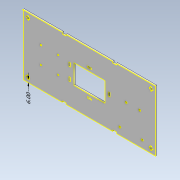
# Autodesk Inventor part: plate_2
Saved by Autodesk Inventor 2022 (Build 260153000, 153)
## iProperties
Created: 2023-04-28
Part Number: plate_2
Material: 一般
Document SubType Name: Modeling
Designer: Johnny Jou
Density: 1 g/cm^3
Appearance: 預設
Author: Johnny Jou
Autodesk Inventor part; units mm, degrees
ref_plane "YZ Plane" through (0, 0, 0) normal (1, 0, 0) x (0, 1, 0)
ref_plane "XZ Plane" through (0, 0, 0) normal (0, 1, 0) x (-1, 0, 0)
ref_plane "XY Plane" through (0, 0, 0) normal (0, 0, 1) x (1, 0, 0)
sketch "草圖1" plane through (0, 0, 0) normal (0, 0, 1) x (1, 0, 0)
  line L0 (0, 0) -> (284, 0)
  line L1 (284, 0) -> (284, -130)
  line L2 (284, -130) -> (0, -130)
  line L3 (0, -130) -> (0, 0)
  dimension "d0" = 284
  dimension "d1" = 130
  constraints: 8 end point, 2 parallel, 1 coincident, 1 horizontal, 1 perpendicular
  measures "d0" distance of L1.end L2.end
  measures "d1" distance of L0.end L1.end
extrude "擠出1" add sketch "草圖1" along normal blind 3
sketch "草圖2" plane through (0, 0, 3) normal (0, 0, 1) x (1, 0, 0)
  line L0 (35, -86.5) -> (78, -86.5)
  line L1 (78, -86.5) -> (78, -43.5)
  line L2 (78, -43.5) -> (35, -43.5)
  line L3 (35, -43.5) -> (35, -86.5)
  circle A0 centre (75, -46.5) radius 1.5
  circle A1 centre (38, -46.5) radius 1.5
  circle A2 centre (75, -83.5) radius 1.5
  circle A3 centre (38, -83.5) radius 1.5
  line L4 (0, 0) -> (0, -130) projected
  line L5 (284, 0) -> (0, 0) projected
  point P0 (74.3802, -81.4068)
  dimension "d44" = 35
  dimension "d45" = 43
  dimension "d46" = 43
  dimension "d47" = 3
  dimension "d48" = 3
  dimension "d49" = 3
  dimension "d50" = 3
  dimension "d51" = 3
  dimension "d52" = 3
  dimension "d53" = 3
  dimension "d54" = 3
  dimension "d55" = 3
  dimension "d56" = 43.5
  constraints: 8 end point, 4 centre point, 3 equal radius, 3 perpendicular
  measures "d44" distance between parallel lines of L4 L3
  measures "d45" distance of L1.end L2.end
  measures "d46" distance of L2.end L0.start
  measures "d47" distance from line of L2 A1.centre
  measures "d48" distance from line of L3 A1.centre
  measures "d49" distance from line of L2 A0.centre
  measures "d50" distance from line of L1 A0.centre
  measures "d51" distance from line of L1 A2.centre
  measures "d52" distance from line of L0 A2.centre
  measures "d53" distance from line of L3 A3.centre
  measures "d54" distance from line of L0 A3.centre
  measures "d55" diameter of A1
  measures "d56" distance between parallel lines of L5 L2
extrude "擠出2" cut sketch "草圖2" against normal up to surface (3 mm away) contours A0 | A1 | A2 | A3
sketch "草圖3" plane through (0, 0, 3) normal (0, 0, 1) x (1, 0, 0)
  line L0 (100.85, -42.4246) -> (100.85, -38)
  line L1 (183.15, -84.8295) -> (183.15, -92)
  line L2 (100.85, -38) -> (183.15, -38)
  line L3 (183.15, -38) -> (183.15, -92)
  line L4 (183.15, -92) -> (100.85, -92)
  line L5 (100.85, -92) -> (100.85, -38)
  line L6 (284, 0) -> (0, 0) projected
  line L7 (284, -130) -> (284, 0) projected
  line L8 (0, 0) -> (284, -130) construction
  line L9 (0, 0) -> (0, -130) projected
  line L10 (0, -130) -> (284, 0) construction
  line L11 (100.85, -38) -> (183.15, -92) construction
  line L12 (183.15, -38) -> (100.85, -92) construction
  line L13 (138, -35.05) -> (146, -35.05)
  line L14 (146, -35.05) -> (146, -38)
  line L15 (146, -38) -> (138, -38)
  line L16 (138, -38) -> (138, -35.05)
  line L17 (138, -92) -> (146, -92)
  line L18 (146, -92) -> (146, -94.95)
  line L19 (146, -94.95) -> (138, -94.95)
  line L20 (138, -94.95) -> (138, -92)
  line L21 (183.15, -61) -> (186.1, -61)
  line L22 (186.1, -61) -> (186.1, -69)
  line L23 (186.1, -69) -> (183.15, -69)
  line L24 (183.15, -69) -> (183.15, -61)
  line L25 (97.9, -48) -> (100.85, -48)
  line L26 (100.85, -48) -> (100.85, -56)
  line L27 (100.85, -56) -> (97.9, -56)
  line L28 (97.9, -56) -> (97.9, -48)
  line L29 (97.9, -75.1961) -> (100.85, -75.1961)
  line L30 (100.85, -75.1961) -> (100.85, -83.1961)
  line L31 (100.85, -83.1961) -> (97.9, -83.1961)
  line L32 (97.9, -83.1961) -> (97.9, -75.1961)
  point P0 (142, -65)
  point P1 (142, -35.05)
  point P2 (142, -65)
  point P3 (186.1, -65)
  point P4 (142, -65)
  dimension "d6" = 54
  dimension "d7" = 82.3
  dimension "d8" = 8
  dimension "d9" = 2.95
  dimension "d10" = 8
  dimension "d11" = 2.95
  dimension "d12" = 8
  dimension "d13" = 2.95
  dimension "d14" = 2.95
  dimension "d15" = 8
  dimension "d16" = 8
  dimension "d17" = 10
  constraints: 60 end point, 12 parallel, 6 horizontal, 6 midpoint, 6 perpendicular, 5 collinear, 2 point on line, 1 horizontal alignment, 1 vertical alignment
  measures "d6" distance between parallel lines of L4 L2
  measures "d7" distance between parallel lines of L5 L3
  measures "d8" distance of L18.end L19.end
  measures "d9" distance of L17.end L18.end
  measures "d10" distance of L13.start L13.end
  measures "d11" distance of L13.end L14.end
  measures "d12" distance of L21.end L22.end
  measures "d13" distance of L21.start L21.end
  measures "d14" distance of L25.start L25.end
  measures "d15" distance of L27.end L25.start
  measures "d16" distance of L31.end L29.start
  measures "d17" distance between parallel lines of L2 L25
extrude "擠出3" cut sketch "草圖3" against normal up to surface (3 mm away) contours L5 L27 L28 L25 | L16 L13 L14 L2 | L5 L31 L32 L29 | L21 L22 L23 L3 | L4 L18 L19 L20
sketch "草圖4" plane through (0, 0, 3) normal (0, 0, 1) x (1, 0, 0)
  line L0 (284, -130) -> (284, 0) projected
  circle A0 centre (249.8545, -61.6059) radius 2
  circle A1 centre (220.8545, -61.6059) radius 2
  circle A2 centre (207.3545, -114.1059) radius 2
  circle A3 centre (255.3545, -114.1059) radius 2
  point P0 (0, 0)
  point P1 (32.4, -26.5)
  dimension "d25" = 48
  dimension "d26" = 5.5
  dimension "d27" = 52.5
  dimension "d28" = 29
  dimension "d29" = 13.5
  dimension "d30" = 52.5
  constraints: 4 centre point
  measures "d25" distance of A3.centre A2.centre
  measures "d26" horizontal distance of A0.centre A3.centre
  measures "d27" vertical distance of A3.centre A0.centre
  measures "d28" distance of A0.centre A1.centre
  measures "d29" horizontal distance of A2.centre A1.centre
  measures "d30" vertical distance of A2.centre A1.centre
extrude "擠出4" cut sketch "草圖4" against normal blind 10
sketch "草圖5" plane through (0, 0, 3) normal (0, 0, 1) x (1, 0, 0)
  line L0 (84, 0) -> (92, 0)
  line L1 (92, 0) -> (92, -2.95)
  line L2 (92, -2.95) -> (84, -2.95)
  line L3 (84, -2.95) -> (84, 0)
  line L4 (192, 0) -> (200, 0)
  line L5 (200, 0) -> (200, -2.95)
  line L6 (200, -2.95) -> (192, -2.95)
  line L7 (192, -2.95) -> (192, 0)
  line L8 (192, -127.05) -> (200, -127.05)
  line L9 (200, -127.05) -> (200, -130)
  line L10 (200, -130) -> (192, -130)
  line L11 (192, -130) -> (192, -127.05)
  line L12 (84, -127.05) -> (92, -127.05)
  line L13 (92, -127.05) -> (92, -130)
  line L14 (92, -130) -> (84, -130)
  line L15 (84, -130) -> (84, -127.05)
  line L16 (284, 0) -> (0, 0) projected
  line L17 (0, -130) -> (284, -130) projected
  line L18 (0, 0) -> (0, -130) projected
  dimension "d33" = 2.95
  dimension "d34" = 8
  dimension "d36" = 2.95
  dimension "d37" = 8
  dimension "d38" = 100
  dimension "d39" = 8
  dimension "d43" = 84
  constraints: 32 end point, 9 collinear, 8 parallel, 4 horizontal, 4 perpendicular
  measures "d33" distance between parallel lines of L2 L0
  measures "d34" distance of L0.start L0.end
  measures "d36" distance between parallel lines of L14 L12
  measures "d37" distance of L13.end L14.end
  measures "d38" distance between parallel lines of L11 L13
  measures "d39" distance of L8.start L8.end
  measures "d43" distance between parallel lines of L18 L3
extrude "擠出5" cut sketch "草圖5" against normal up to surface (3 mm away)
sketch "草圖6" plane through (0, 0, 3) normal (0, 0, 1) x (1, 0, 0)
  line L0 (8.525, -6) -> (11.475, -6)
  line L1 (11.475, -6) -> (11.475, -14)
  line L2 (11.475, -14) -> (8.525, -14)
  line L3 (8.525, -14) -> (8.525, -6)
  line L4 (6, -8.525) -> (14, -8.525)
  line L5 (14, -8.525) -> (14, -11.475)
  line L6 (14, -11.475) -> (6, -11.475)
  line L7 (6, -11.475) -> (6, -8.525)
  line L8 (6, -8.525) -> (14, -11.475) construction
  line L9 (14, -8.525) -> (6, -11.475) construction
  line L10 (8.525, -14) -> (11.475, -6) construction
  line L11 (11.475, -14) -> (8.525, -6) construction
  line L12 (84, 0) -> (0, 0) construction
  line L13 (0, 0) -> (0, -130) construction
  point P0 (10, -10)
  point P1 (8.525, -11.475)
  point P2 (11.475, -11.475)
  point P3 (11.475, -8.525)
  point P4 (8.525, -8.525)
  dimension "d57" = 8
  dimension "d58" = 8
  dimension "d59" = 2.95
  dimension "d60" = 2.95
  dimension "d61" = 6
  dimension "d62" = 6
  constraints: 24 end point, 4 parallel, 2 horizontal, 2 midpoint, 2 perpendicular
  measures "d57" distance of L4.start L4.end
  measures "d58" distance of L0.end L1.end
  measures "d59" distance of L0.start L0.end
  measures "d60" distance of L4.end L5.end
  measures "d61" distance between parallel lines of L12 L0
  measures "d62" distance between parallel lines of L13 L7
extrude "擠出6" cut sketch "草圖6" against normal up to surface (3 mm away)
pattern_linear "矩形陣列1" count 2 spacing 110 along (0, -1, 0) count 2 spacing 264 along (1, 0, 0) of "擠出6"
sketch "草圖7" plane through (0, 0, 3) normal (0, 0, 1) x (1, 0, 0)
  line L0 (108.85, -44) -> (175.15, -44)
  line L1 (175.15, -44) -> (175.15, -86)
  line L2 (175.15, -86) -> (108.85, -86)
  line L3 (108.85, -86) -> (108.85, -44)
  line L4 (146, -38) -> (138, -38) projected
  line L5 (138, -92) -> (146, -92) projected
  line L6 (183.15, -69) -> (183.15, -61) projected
  line L7 (100.85, -48) -> (100.85, -56) projected
  point P0 (0, 0)
  dimension "d74" = 6
  dimension "d75" = 6
  dimension "d76" = 8
  dimension "d77" = 8
  constraints: 8 end point, 2 parallel, 1 horizontal, 1 perpendicular
  measures "d74" distance between parallel lines of L0 L4
  measures "d75" distance between parallel lines of L5 L2
  measures "d76" distance between parallel lines of L6 L1
  measures "d77" distance between parallel lines of L7 L3
extrude "擠出7" cut sketch "草圖7" against normal blind 10
sketch "草圖8" plane through (0, 0, 3) normal (0, 0, 1) x (1, 0, 0)
  line L0 (175.15, -44) -> (175.15, -86) projected
  line L1 (175.15, -86) -> (108.85, -86) projected
  line L2 (108.85, -86) -> (108.85, -44) projected
  line L3 (108.85, -44) -> (175.15, -44) projected
  line L4 (272.525, -116) -> (275.475, -116) projected
  line L5 (275.475, -116) -> (275.475, -118.525) projected
  line L6 (275.475, -118.525) -> (278, -118.525) projected
  line L7 (278, -118.525) -> (278, -121.475) projected
  line L8 (278, -121.475) -> (275.475, -121.475) projected
  line L9 (275.475, -121.475) -> (275.475, -124) projected
  line L10 (275.475, -124) -> (272.525, -124) projected
  line L11 (272.525, -124) -> (272.525, -121.475) projected
  line L12 (272.525, -121.475) -> (270, -121.475) projected
  line L13 (270, -121.475) -> (270, -118.525) projected
  line L14 (270, -118.525) -> (272.525, -118.525) projected
  line L15 (272.525, -118.525) -> (272.525, -116) projected
  line L16 (272.525, -6) -> (275.475, -6) projected
  line L17 (275.475, -6) -> (275.475, -8.525) projected
  line L18 (275.475, -8.525) -> (278, -8.525) projected
  line L19 (278, -8.525) -> (278, -11.475) projected
  line L20 (278, -11.475) -> (275.475, -11.475) projected
  line L21 (275.475, -11.475) -> (275.475, -14) projected
  line L22 (275.475, -14) -> (272.525, -14) projected
  line L23 (272.525, -14) -> (272.525, -11.475) projected
  line L24 (272.525, -11.475) -> (270, -11.475) projected
  line L25 (270, -11.475) -> (270, -8.525) projected
  line L26 (270, -8.525) -> (272.525, -8.525) projected
  line L27 (272.525, -8.525) -> (272.525, -6) projected
  line L28 (8.525, -116) -> (11.475, -116) projected
  line L29 (11.475, -116) -> (11.475, -118.525) projected
  line L30 (11.475, -118.525) -> (14, -118.525) projected
  line L31 (14, -118.525) -> (14, -121.475) projected
  line L32 (14, -121.475) -> (11.475, -121.475) projected
  line L33 (11.475, -121.475) -> (11.475, -124) projected
  line L34 (11.475, -124) -> (8.525, -124) projected
  line L35 (8.525, -124) -> (8.525, -121.475) projected
  line L36 (8.525, -121.475) -> (6, -121.475) projected
  line L37 (6, -121.475) -> (6, -118.525) projected
  line L38 (6, -118.525) -> (8.525, -118.525) projected
  line L39 (8.525, -118.525) -> (8.525, -116) projected
  line L40 (8.525, -6) -> (11.475, -6) projected
  line L41 (11.475, -6) -> (11.475, -8.525) projected
  line L42 (11.475, -8.525) -> (14, -8.525) projected
  line L43 (14, -8.525) -> (14, -11.475) projected
  line L44 (14, -11.475) -> (11.475, -11.475) projected
  line L45 (11.475, -11.475) -> (11.475, -14) projected
  line L46 (11.475, -14) -> (8.525, -14) projected
  line L47 (8.525, -14) -> (8.525, -11.475) projected
  line L48 (8.525, -11.475) -> (6, -11.475) projected
  line L49 (6, -11.475) -> (6, -8.525) projected
  line L50 (6, -8.525) -> (8.525, -8.525) projected
  line L51 (8.525, -8.525) -> (8.525, -6) projected
  line L52 (192, -2.95) -> (192, 0) projected
  line L53 (192, 0) -> (92, 0) projected
  line L54 (92, 0) -> (92, -2.95) projected
  line L55 (92, -2.95) -> (84, -2.95) projected
  line L56 (84, -2.95) -> (84, 0) projected
  line L57 (84, 0) -> (0, 0) projected
  line L58 (0, 0) -> (0, -130) projected
  line L59 (0, -130) -> (84, -130) projected
  line L60 (84, -130) -> (84, -127.05) projected
  line L61 (84, -127.05) -> (92, -127.05) projected
  line L62 (92, -127.05) -> (92, -130) projected
  line L63 (92, -130) -> (192, -130) projected
  line L64 (192, -130) -> (192, -127.05) projected
  line L65 (192, -127.05) -> (200, -127.05) projected
  line L66 (200, -127.05) -> (200, -130) projected
  line L67 (200, -130) -> (284, -130) projected
  line L68 (284, -130) -> (284, 0) projected
  line L69 (284, 0) -> (200, 0) projected
  line L70 (200, 0) -> (200, -2.95) projected
  line L71 (200, -2.95) -> (192, -2.95) projected
  circle A0 centre (207.3545, -114.1059) radius 2 projected
  circle A1 centre (220.8545, -61.6059) radius 2 projected
  circle A2 centre (249.8545, -61.6059) radius 2 projected
  circle A3 centre (255.3545, -114.1059) radius 2 projected
  line L72 (146, -92) -> (146, -94.95) projected
  line L73 (146, -94.95) -> (138, -94.95) projected
  line L74 (138, -94.95) -> (138, -92) projected
  line L75 (138, -92) -> (146, -92) projected
  line L76 (138, -38) -> (138, -35.05) projected
  line L77 (138, -35.05) -> (146, -35.05) projected
  line L78 (146, -35.05) -> (146, -38) projected
  line L79 (146, -38) -> (138, -38) projected
  line L80 (97.9, -83.1961) -> (97.9, -75.1961) projected
  line L81 (97.9, -75.1961) -> (100.85, -75.1961) projected
  line L82 (100.85, -75.1961) -> (100.85, -83.1961) projected
  line L83 (100.85, -83.1961) -> (97.9, -83.1961) projected
  line L84 (183.15, -61) -> (186.1, -61) projected
  line L85 (186.1, -61) -> (186.1, -69) projected
  line L86 (186.1, -69) -> (183.15, -69) projected
  line L87 (183.15, -69) -> (183.15, -61) projected
  line L88 (97.9, -56) -> (97.9, -48) projected
  line L89 (97.9, -48) -> (100.85, -48) projected
  line L90 (100.85, -48) -> (100.85, -56) projected
  line L91 (100.85, -56) -> (97.9, -56) projected
  circle A4 centre (75, -83.5) radius 1.5 projected
  circle A5 centre (38, -46.5) radius 1.5 projected
  circle A6 centre (38, -83.5) radius 1.5 projected
  circle A7 centre (75, -46.5) radius 1.5 projected
